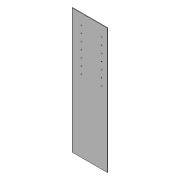
# Autodesk Inventor part: Cut_B
Saved by Autodesk Inventor 2020 (Build 240168000, 168)
## iProperties
Created: 2021-12-11
Part Number: Cut_B
Material: Generic
Document SubType Name: Modeling
Designer: magnarecta
Density: 1 g/cm^3
Appearance: Default
Author: magnarecta
Autodesk Inventor part; units mm, degrees
ref_plane "YZ Plane" through (0, 0, 0) normal (1, 0, 0) x (0, 1, 0)
ref_plane "XZ Plane" through (0, 0, 0) normal (0, 1, 0) x (-1, 0, 0)
ref_plane "XY Plane" through (0, 0, 0) normal (0, 0, 1) x (1, 0, 0)
sketch "スケッチ1" plane through (0, 0, 0) normal (0, 0, 1) x (1, 0, 0)
  line L0 (99, -354) -> (-99, -354)
  line L1 (-99, -354) -> (-99, 354)
  line L2 (-99, 354) -> (99, 354)
  line L3 (99, 354) -> (99, -354)
  line L4 (99, -354) -> (-99, 354) construction
  line L5 (-99, -354) -> (99, 354) construction
  point P0 (0, 0)
  dimension "d0" = 198
  dimension "d1" = 708
  constraints: 12 end point, 2 midpoint, 2 parallel, 1 horizontal, 1 perpendicular
  measures "d0" distance of L1.end L2.end
  measures "d1" distance of L0.end L1.end
extrude "押し出し1" add sketch "スケッチ1" along normal blind 3
sketch "スケッチ2" plane through (0, 0, 3) normal (0, 0, 1) x (1, 0, 0)
  line L0 (99, -354) -> (99, 354) projected
  line L1 (-99, -354) -> (99, -354) projected
  line L2 (99, 354) -> (-99, 354) projected
  point P0 (0, 0)
  point P1 (67.5, 294)
  point P2 (-47.5, 294)
  point P3 (67.5, 254)
  point P4 (-47.5, 254)
  point P5 (67.5, 214)
  point P6 (-47.5, 214)
  point P7 (67.5, 174)
  point P8 (-47.5, 174)
  point P9 (67.5, 134)
  point P10 (-47.5, 134)
  point P11 (67.5, 94)
  point P12 (-47.5, 94)
  point P13 (67.5, 54)
  point P14 (-47.5, 54)
  dimension "d4" = 115
  dimension "d7" = 40
  dimension "d12" = 47.5
  dimension "d21" = 60
  constraints: 1 horizontal alignment, 1 vertical, 12 other
  measures "d4" distance of point (67.5, 294) point (-47.5, 294)
  measures "d7" distance of point (67.5, 294) point (67.5, 254)
  measures "d12" horizontal distance of point (0, 0) point (-47.5, 294)
  measures "d21" distance from line of point (67.5, 294) L2
hole "穴1" at (67.5, 294, 3) at (-47.5, 294, 3) at (67.5, 254, 3) at (-47.5, 254, 3) at (67.5, 214, 3) at (-47.5, 214, 3) at (67.5, 174, 3) at (-47.5, 174, 3) at (67.5, 134, 3) at (-47.5, 134, 3) at (67.5, 94, 3) at (-47.5, 94, 3) at (67.5, 54, 3) at (-47.5, 54, 3) direction (0, 0, -1) diameter 4.2 end through all
